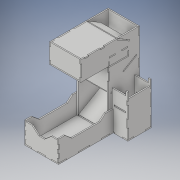
# Autodesk Inventor part: fulltowerv2
Saved by Autodesk Inventor 2017 (Build 210142000, 142)
## iProperties
Created: 2017-03-30
Part Number: fulltowerv2
Material: Generic
Document SubType Name: Modeling
Designer: bearb
Density: 1 g/cm^3
Appearance: Default
Author: bearb
Autodesk Inventor part; units mm, degrees
ref_plane "YZ Plane" through (0, 0, 0) normal (1, 0, 0) x (0, 1, 0)
ref_plane "XZ Plane" through (0, 0, 0) normal (0, 1, 0) x (-1, 0, 0)
ref_plane "XY Plane" through (0, 0, 0) normal (0, 0, 1) x (1, 0, 0)
sketch "Sketch1" plane through (0, 0, 0) normal (1, 0, 0) x (0, 1, 0)
  line L0 (254, 3.81) -> (254, 101.6)
  line L1 (190.5, 101.6) -> (190.5, 34.798)
  line L2 (192.0504, 98.044) -> (212.3704, 98.044) construction
  line L3 (212.3704, 98.044) -> (212.3704, 38.354) construction
  line L4 (212.3704, 38.354) -> (192.0504, 38.354) construction
  line L5 (192.0504, 38.354) -> (192.0504, 98.044) construction
  line L6 (190.5, 101.6) -> (203.2, 101.6)
  line L7 (203.2, 101.6) -> (203.2, 98.044)
  line L8 (203.2, 98.044) -> (190.5, 98.044)
  line L9 (190.5, 98.044) -> (190.5, 101.6)
  line L10 (190.5, 34.798) -> (203.2, 34.798)
  line L11 (203.2, 34.798) -> (203.2, 38.354)
  line L12 (203.2, 38.354) -> (190.5, 38.354)
  line L13 (190.5, 38.354) -> (190.5, 34.798)
  line L14 (190.5, 101.6) -> (186.69, 101.6)
  line L15 (186.69, 101.6) -> (186.69, 34.798)
  line L16 (186.69, 34.798) -> (190.5, 34.798)
  line L17 (212.3704, 38.354) -> (216.1804, 38.354)
  line L18 (216.1804, 38.354) -> (216.1804, 57.404)
  line L19 (216.1804, 57.404) -> (212.3704, 57.404)
  line L20 (212.3704, 57.404) -> (212.3704, 38.354)
  line L21 (212.3704, 98.044) -> (216.1804, 98.044)
  line L22 (216.1804, 98.044) -> (216.1804, 78.994)
  line L23 (216.1804, 78.994) -> (212.3704, 78.994)
  line L24 (212.3704, 78.994) -> (212.3704, 98.044)
  line L25 (231.3686, 31.75) -> (254, 70.9487)
  line L26 (250.9204, 72.7267) -> (228.289, 33.528)
  line L27 (228.289, 33.528) -> (231.3686, 31.75)
  line L28 (254, 70.9487) -> (250.9204, 72.7267)
  line L29 (179.2898, 10.16) -> (153.8898, 54.1541)
  line L30 (153.8898, 54.1541) -> (150.8102, 52.3761)
  line L31 (150.8102, 52.3761) -> (176.2102, 8.382)
  line L32 (176.2102, 8.382) -> (179.2898, 10.16)
  line L33 (114.3, 91.44) -> (85.2445, 41.1145)
  line L34 (85.2445, 41.1145) -> (82.165, 42.8925)
  line L35 (82.165, 42.8925) -> (111.2204, 93.218)
  line L36 (111.2204, 93.218) -> (114.3, 91.44)
  line L37 (9.525, 94.4269) -> (57.15, 11.938)
  line L38 (57.15, 11.938) -> (54.0704, 10.16)
  line L39 (54.0704, 10.16) -> (6.4454, 92.6489)
  line L40 (6.4454, 92.6489) -> (9.525, 94.4269)
  line L41 (254, 177.8) -> (250.19, 177.8)
  line L42 (250.19, 177.8) -> (250.19, 165.1)
  line L43 (250.19, 165.1) -> (254, 165.1)
  line L44 (254, 177.8) -> (254, 190.5)
  line L45 (254, 165.1) -> (254, 127)
  line L46 (254, 127) -> (250.19, 127)
  line L47 (250.19, 127) -> (250.19, 114.3)
  line L48 (250.19, 114.3) -> (254, 114.3)
  line L49 (254, 101.6) -> (254, 114.3)
  line L50 (254, 127) -> (254, 165.1)
  line L51 (228.6, 0) -> (228.6, 3.81)
  line L52 (228.6, 3.81) -> (254, 3.81)
  line L53 (228.6, 0) -> (165.1, 0)
  line L54 (165.1, 0) -> (165.1, 3.81)
  line L55 (165.1, 3.81) -> (139.7, 3.81)
  line L56 (139.7, 3.81) -> (139.7, 0)
  line L57 (139.7, 0) -> (114.3, 0)
  line L58 (114.3, 0) -> (114.3, 3.81)
  line L59 (114.3, 3.81) -> (88.9, 3.81)
  line L60 (88.9, 3.81) -> (88.9, 0)
  line L61 (88.9, 0) -> (50.8, 0)
  line L62 (50.8, 0) -> (50.8, 3.81)
  line L63 (50.8, 3.81) -> (25.4, 3.81)
  line L64 (25.4, 3.81) -> (25.4, 0)
  line L65 (0, 0) -> (25.4, 0)
  line L66 (50.8, 0) -> (88.9, 0)
  line L67 (114.3, 0) -> (139.7, 0)
  line L68 (165.1, 0) -> (228.6, 0)
  line L69 (186.69, 101.6) -> (173.99, 101.6)
  line L70 (173.99, 101.6) -> (173.99, 97.79)
  line L71 (173.99, 97.79) -> (148.59, 97.79)
  line L72 (148.59, 97.79) -> (148.59, 101.6)
  line L73 (190.5, 101.6) -> (173.99, 101.6)
  line L74 (148.59, 101.6) -> (0, 101.6)
  line L75 (0, 101.6) -> (0, 88.9)
  line L76 (0, 0) -> (0, 12.7)
  line L77 (0, 12.7) -> (3.81, 12.7)
  line L78 (0, 88.9) -> (3.81, 88.9)
  line L79 (3.81, 88.9) -> (3.81, 12.7)
  line L80 (0, 101.6) -> (0, 88.9)
  line L81 (0, 12.7) -> (0, 0)
  line L82 (190.5, 190.5) -> (190.5, 177.8)
  line L83 (190.5, 177.8) -> (194.31, 177.8)
  line L84 (194.31, 177.8) -> (194.31, 165.1)
  line L85 (194.31, 165.1) -> (190.5, 165.1)
  line L86 (190.5, 165.1) -> (190.5, 127)
  line L87 (190.5, 127) -> (194.31, 127)
  line L88 (194.31, 127) -> (194.31, 114.3)
  line L89 (194.31, 114.3) -> (190.5, 114.3)
  line L90 (190.5, 101.6) -> (190.5, 114.3)
  line L91 (190.5, 127) -> (190.5, 165.1)
  line L92 (190.5, 177.8) -> (190.5, 190.5)
  line L93 (190.5, 190.5) -> (203.2, 190.5)
  line L94 (203.2, 190.5) -> (203.2, 186.69)
  line L95 (203.2, 186.69) -> (241.3, 186.69)
  line L96 (241.3, 186.69) -> (241.3, 190.5)
  line L97 (190.5, 190.5) -> (203.2, 190.5)
  line L98 (241.3, 190.5) -> (254, 190.5)
  dimension "d0" = 254
  dimension "d2" = 66.802
  dimension "d4" = 20.32
  dimension "d5" = 59.69
  dimension "d6" = 88.9
  dimension "d7" = 12.7
  dimension "d8" = 3.556
  dimension "d9" = 12.7
  dimension "d10" = 3.556
  dimension "d12" = 3.81
  dimension "d13" = 3.81
  dimension "d14" = 19.05
  dimension "d15" = 3.81
  dimension "d16" = 19.05
  dimension "d18" = 3.556
  dimension "d21" = 3.556
  dimension "d22" = 3.556
  dimension "d23" = 3.556
  dimension "d27" = 50.8
  dimension "d30" = 95.25
  dimension "d34" = 3.81
  dimension "d37" = 12.7
  dimension "d38" = 38.1
  dimension "d39" = 3.81
  dimension "d40" = 12.7
  dimension "d43" = 3.81
  dimension "d45" = 3.81
  dimension "d46" = 25.4
  dimension "d47" = 25.4
  dimension "d48" = 25.4
  dimension "d49" = 38.1
  dimension "d50" = 25.4
  dimension "d52" = 12.7
  dimension "d53" = 3.81
  dimension "d54" = 25.4
  dimension "d55" = 12.7
  dimension "d56" = 12.7
  dimension "d57" = 3.81
  dimension "d160" = 12.7
  dimension "d161" = 3.81
  dimension "d162" = 12.7
  dimension "d163" = 38.1
  dimension "d164" = 12.7
  dimension "d165" = 12.7
  dimension "d166" = 3.81
  constraints: 198 end point, 66 perpendicular, 25 parallel, 13 horizontal, 8 point on line, 4 vertical
  measures "d0" distance of L74.end L0.end
  measures "d2" distance of L1.start L1.end
  measures "d4" distance of L3.end L4.end
  measures "d5" distance of L2.end L3.end
  measures "d6" distance of L1.start L82.start
  measures "d7" distance of L7.end L8.end
  measures "d8" distance of L6.end L7.end
  measures "d9" distance of L12.end L11.end
  measures "d10" distance of L11.end L10.end
  measures "d12" distance of L1.start L14.end
  measures "d13" distance of L19.end L18.end
  measures "d14" distance of L18.end L17.end
  measures "d15" distance of L22.end L23.end
  measures "d16" distance of L21.end L22.end
  measures "d18" distance between parallel lines of L26 L25
  measures "d21" distance of L29.end L30.end
  measures "d22" distance of L33.end L34.end
  measures "d23" distance of L37.end L38.end
  measures "d27" distance between parallel lines of L30 L32
  measures "d30" distance between parallel lines of L40 L38
  measures "d34" distance of L43.end L42.end
  measures "d37" distance between parallel lines of L43 L41
  measures "d38" distance of L43.end L45.end
  measures "d39" distance of L45.end L46.end
  measures "d40" distance of L46.end L47.end
  measures "d43" distance of L51.start L51.end
  measures "d45" distance of L53.end L54.end
  measures "d46" distance of L54.end L55.end
  measures "d47" distance of L56.end L57.end
  measures "d48" distance of L58.end L59.end
  measures "d49" distance of L60.end L61.end
  measures "d50" distance of L62.end L63.end
  measures "d52" distance of L14.end L69.end
  measures "d53" distance of L69.end L70.end
  measures "d54" distance of L70.end L71.end
  measures "d55" distance of L74.end L75.end
  measures "d56" distance of L65.start L76.end
  measures "d57" distance of L76.end L77.end
  measures "d160" distance of L82.start L82.end
  measures "d161" distance of L82.end L83.end
  measures "d162" distance of L83.end L84.end
  measures "d163" distance of L85.end L86.end
  measures "d164" distance of L87.end L88.end
  measures "d165" distance of L82.start L93.end
  measures "d166" distance of L93.end L94.end
extrude "Extrusion1" add sketch "Sketch1" along normal blind 3.81 contours L52 L51 L53 L54 L55 L56 L57 L58 L59 L60 L61 L62 L63 L64 L65 L76 L77 L79 L78 L75 L74 L72 L71 L70 L69 L15 L16 L10 L11 L12 L1 L8 L7 L6 L90 L89 L88 L87 L86 L85 L84 L83 L82 L93 L94 L95 L96 L98 L44 L41 L42 L43 L45 L46 L47 L48 L49 L0
sketch "Sketch2" plane through (0, 228.6, 3.81) normal (0, 0, -1) x (-1, 0, 0)
  line L0 (0, 25.4) -> (-3.81, 25.4) projected
  line L1 (0, 25.4) -> (-3.81, 25.4)
  line L2 (0, 0) -> (-3.81, 0) projected
  line L3 (-3.81, 25.4) -> (-3.81, 0)
  line L4 (-3.81, 0) -> (0, 0)
  line L5 (0, 0) -> (0, -63.5)
  line L6 (0, -63.5) -> (-3.81, -63.5) projected
  line L7 (0, -63.5) -> (-3.81, -63.5)
  line L8 (0, -88.9) -> (-3.81, -88.9) projected
  line L9 (-3.81, -63.5) -> (-3.81, -88.9)
  line L10 (-3.81, -88.9) -> (0, -88.9)
  line L11 (0, -88.9) -> (0, -114.3)
  line L12 (0, -114.3) -> (-3.81, -114.3) projected
  line L13 (0, -114.3) -> (-3.81, -114.3)
  line L14 (-3.81, -139.7) -> (-3.81, -114.3) projected
  line L15 (-3.81, -114.3) -> (-3.81, -139.7)
  line L16 (-3.81, -139.7) -> (0, -139.7)
  line L17 (0, -139.7) -> (0, -177.8)
  line L18 (0, -177.8) -> (-3.81, -177.8) projected
  line L19 (0, -177.8) -> (-3.81, -177.8)
  line L20 (-3.81, -177.8) -> (-3.81, -203.2)
  line L21 (0, -203.2) -> (-3.81, -203.2) projected
  line L22 (-3.81, -203.2) -> (0, -203.2)
  line L23 (0, -228.6) -> (-3.81, -228.6) projected
  line L24 (0, -203.2) -> (0, -215.9)
  line L25 (6.35, -228.6) -> (93.98, -228.6)
  line L26 (0, 25.4) -> (-3.81, 25.4) projected
  line L27 (0, 25.4) -> (93.98, 25.4)
  line L28 (93.98, 25.4) -> (97.79, 25.4)
  line L29 (97.79, 25.4) -> (97.79, 0)
  line L30 (97.79, 0) -> (93.98, 0)
  line L31 (93.98, 0) -> (93.98, -63.5)
  line L32 (93.98, -63.5) -> (97.79, -63.5)
  line L33 (97.79, -63.5) -> (97.79, -88.9)
  line L34 (97.79, -88.9) -> (93.98, -88.9)
  line L35 (93.98, -88.9) -> (93.98, -114.3)
  line L36 (93.98, -114.3) -> (97.79, -114.3)
  line L37 (97.79, -114.3) -> (97.79, -139.7)
  line L38 (97.79, -139.7) -> (93.98, -139.7)
  line L39 (93.98, -139.7) -> (93.98, -177.8)
  line L40 (93.98, -177.8) -> (97.79, -177.8)
  line L41 (97.79, -177.8) -> (97.79, -203.2)
  line L42 (97.79, -203.2) -> (93.98, -203.2)
  line L43 (93.98, -203.2) -> (93.98, -228.6)
  line L44 (0, -80.01) -> (0, -228.6) projected
  line L45 (6.35, -228.6) -> (6.35, -215.9)
  line L46 (6.35, -215.9) -> (0, -215.9)
  point P0 (0, -222.25)
  dimension "d62" = 3.81
  dimension "d74" = 93.98
  dimension "d294" = 12.7
  dimension "d295" = 6.35
  constraints: 72 end point, 18 perpendicular, 13 point on line, 6 collinear, 3 horizontal, 1 vertical
  measures "d62" distance of L27.end L28.end
  measures "d74" distance of L0.start L27.end
  measures "d294" distance of L25.start L45.end
  measures "d295" distance of L24.end L45.end
extrude "Extrusion2" add sketch "Sketch2" along normal blind 3.81 separate body contours L27 L28 L29 L30 L31 L32 L33 L34 L35 L36 L37 L38 L39 L40 L41 L42 L43 L25 L45 L46 L24 L44 L17 L11 L8 L9 L6 L5 L2 L3 L0 | L44 L16 L14 L12
ref_plane "Work Plane1" through (-46.99, 0, 0) normal (-1, 0, 0) x (0, 0, 1)
mirror "Mirror1" about plane through (-46.99, 0, 0) normal (-1, 0, 0) bodies 1 separate body
sketch "Sketch5" plane through (-97.79, 54.0704, 10.16) normal (0, 0.8660254, 0.5) x (1, 0, 0)
  line L0 (97.79, 0) -> (101.6, 0) projected
  line L1 (101.6, 0) -> (97.79, 0)
  line L2 (97.79, 0) -> (97.79, 6.35)
  line L3 (97.79, 6.35) -> (3.81, 6.35)
  line L4 (3.81, 6.35) -> (3.81, 0)
  line L5 (3.81, 0) -> (0, 0) projected
  line L6 (3.81, 0) -> (0, 0)
  line L7 (0, 0) -> (0, -95.25)
  line L8 (0, -95.25) -> (3.81, -95.25)
  line L9 (3.81, -95.25) -> (3.81, -101.6)
  line L10 (3.81, -101.6) -> (97.79, -101.6)
  line L11 (97.79, -101.6) -> (97.79, -95.25)
  line L12 (97.79, -95.25) -> (101.6, -95.25) projected
  line L13 (97.79, -95.25) -> (101.6, -95.25)
  line L14 (101.6, 0) -> (101.6, -95.25) projected
  line L15 (101.6, -95.25) -> (101.6, 0)
  dimension "d84" = 6.35
  dimension "d85" = 93.98
  dimension "d86" = 3.81
  dimension "d87" = 6.35
  dimension "d88" = 93.98
  dimension "d89" = 6.35
  dimension "d90" = 3.81
  constraints: 24 end point, 5 perpendicular, 3 point on line, 2 collinear, 1 horizontal
  measures "d84" distance of L0.start L2.end
  measures "d85" distance of L2.end L3.end
  measures "d86" distance of L4.end L5.end
  measures "d87" distance of L8.end L9.end
  measures "d88" distance of L9.end L10.end
  measures "d89" distance of L10.end L11.end
  measures "d90" distance of L11.end L12.end
extrude "Extrusion3" add sketch "Sketch5" along normal blind 3.81 separate body
sketch "Sketch7" plane through (0, 111.2204, 93.218) normal (0, 0.8660254, -0.5) x (1, 0, 0)
  line L0 (3.81, 58.1109) -> (3.81, 0) projected
  line L1 (3.81, 0) -> (3.81, 58.1109)
  line L2 (0, 58.1109) -> (3.81, 58.1109) projected
  line L3 (3.81, 58.1109) -> (0, 58.1109)
  line L4 (0, 0) -> (3.81, 0) projected
  line L5 (3.81, 0) -> (0, 0)
  line L6 (0, 58.1109) -> (0, 64.4609)
  line L7 (0, 64.4609) -> (-93.98, 64.4609)
  line L8 (-97.79, 58.1109) -> (-97.79, 0) projected
  line L9 (-97.79, 58.1109) -> (-97.79, 0)
  line L10 (-97.79, 0) -> (-93.98, 0)
  line L11 (-93.98, 58.1109) -> (-97.79, 58.1109) projected
  line L12 (-97.79, 58.1109) -> (-93.98, 58.1109)
  line L13 (-93.98, 58.1109) -> (-93.98, 64.4609)
  line L14 (0, 0) -> (0, -6.35)
  line L15 (0, -6.35) -> (-93.98, -6.35)
  line L16 (-93.98, -6.35) -> (-93.98, 0)
  point P0 (0, 136.3394)
  dimension "d100" = 3.81
  dimension "d101" = 3.81
  dimension "d102" = 6.35
  dimension "d103" = 93.98
  dimension "d104" = 3.81
  dimension "d105" = 6.35
  dimension "d106" = 93.98
  constraints: 24 end point, 3 collinear, 3 perpendicular, 2 vertical, 1 horizontal
  measures "d100" distance of L0.start L2.start
  measures "d101" distance of L0.end L4.start
  measures "d102" distance of L2.start L6.end
  measures "d103" distance of L6.end L7.end
  measures "d104" distance of L8.end L10.end
  measures "d105" distance of L4.start L14.end
  measures "d106" distance of L14.end L15.end
extrude "Extrusion4" add sketch "Sketch7" along normal blind 3.81 separate body
sketch "Sketch8" plane through (0, 150.8102, 52.3761) normal (0, 0.8660254, 0.5) x (1, 0, 0)
  line L0 (3.81, 50.8) -> (3.81, 0) projected
  line L1 (3.81, 0) -> (3.81, 50.8)
  line L2 (0, 50.8) -> (3.81, 50.8) projected
  line L3 (3.81, 50.8) -> (0, 50.8)
  line L4 (0, 0) -> (3.81, 0) projected
  line L5 (3.81, 0) -> (0, 0)
  line L6 (-97.79, 50.8) -> (-97.79, 0) projected
  line L7 (-97.79, 0) -> (-97.79, 50.8)
  line L8 (-97.79, 50.8) -> (-93.98, 50.8)
  line L9 (-93.98, 0) -> (-97.79, 0) projected
  line L10 (-97.79, 0) -> (-93.98, 0)
  line L11 (0, 50.8) -> (0, 53.34)
  line L12 (0, 53.34) -> (-93.98, 53.34)
  line L13 (-93.98, 53.34) -> (-93.98, 50.8)
  line L14 (0, 0) -> (0, -6.35)
  line L15 (0, -6.35) -> (-93.98, -6.35)
  line L16 (-93.98, -6.35) -> (-93.98, 0)
  point P0 (0, -30.0461)
  dimension "d109" = 3.81
  dimension "d110" = 3.81
  dimension "d111" = 3.81
  dimension "d112" = 3.81
  dimension "d113" = 2.54
  dimension "d114" = 93.98
  dimension "d115" = 6.35
  dimension "d116" = 93.98
  constraints: 24 end point, 3 collinear, 3 perpendicular, 3 vertical, 1 horizontal
  measures "d109" distance of L0.start L2.start
  measures "d110" distance of L0.end L4.start
  measures "d111" distance of L6.start L8.end
  measures "d112" distance of L6.end L9.start
  measures "d113" distance of L2.start L11.end
  measures "d114" distance of L11.end L12.end
  measures "d115" distance of L4.start L14.end
  measures "d116" distance of L14.end L15.end
extrude "Extrusion5" add sketch "Sketch8" along normal blind 3.81 separate body
sketch "Sketch9" plane through (0, 186.69, 101.6) normal (0, 1, 0) x (1, 0, 0)
  line L0 (3.81, 66.802) -> (3.81, 0) projected
  line L1 (0, 66.802) -> (3.81, 66.802) projected
  line L2 (3.81, 0) -> (3.81, 66.802)
  line L3 (3.81, 66.802) -> (-97.79, 66.802)
  line L4 (-93.98, 0) -> (-97.79, 0) projected
  line L5 (-97.79, 66.802) -> (-97.79, 0)
  line L6 (-97.79, 0) -> (3.81, 0)
  point P0 (0, 101.6)
  dimension "d119" = 101.6
  dimension "d120" = 101.6
  constraints: 8 end point, 2 collinear, 1 vertical
  measures "d119" distance of L0.start L3.end
  measures "d120" distance of L4.end L0.end
extrude "Extrusion6" add sketch "Sketch9" along normal blind 3.81 separate body
sketch "Sketch10" plane through (0, 190.5, 98.044) normal (0, 0, 1) x (1, 0, 0)
  line L0 (3.81, 0) -> (3.81, 12.7) projected
  line L1 (3.81, 12.7) -> (3.81, 0)
  line L2 (3.81, 0) -> (-97.79, 0)
  line L3 (0, 0) -> (3.81, 0) projected
  line L4 (-97.79, 0) -> (-97.79, 12.7)
  line L5 (-97.79, 12.7) -> (3.81, 12.7)
  line L6 (-93.98, 12.7) -> (-97.79, 12.7) projected
  point P0 (0, -190.5)
  dimension "d123" = 101.6
  dimension "d124" = 101.6
  constraints: 8 end point, 2 collinear, 1 perpendicular, 1 vertical
  measures "d123" distance of L0.start L2.end
  measures "d124" distance of L4.end L0.end
extrude "Extrusion7" add sketch "Sketch10" along normal blind 3.556 separate body
sketch "Sketch13" plane through (0, 186.69, 34.798) normal (0, 0, 1) x (1, 0, 0)
  line L0 (0, 16.51) -> (3.81, 16.51) projected
  line L1 (3.81, 3.81) -> (-97.79, 3.81) projected
  line L2 (3.81, 3.81) -> (-97.79, 3.81)
  line L3 (-97.79, 3.81) -> (-97.79, 16.51)
  line L4 (-97.79, 16.51) -> (3.81, 16.51)
  line L5 (3.81, 16.51) -> (3.81, 3.81)
  dimension "d136" = 12.7
  dimension "d137" = 101.6
  constraints: 8 end point, 1 collinear, 1 horizontal, 1 perpendicular, 1 point on line, 1 vertical
  measures "d136" distance of L1.end L3.end
  measures "d137" distance of L3.end L0.end
extrude "Extrusion8" add sketch "Sketch13" along normal blind 3.556 separate body
sketch "Sketch14" plane through (0, 212.3704, 57.404) normal (0, 1, 0) x (1, 0, 0)
  line L0 (3.81, 19.05) -> (3.81, 0) projected
  line L1 (3.81, 0) -> (3.81, 19.05)
  line L2 (3.81, 19.05) -> (-97.79, 19.05)
  line L3 (-97.79, 0) -> (-97.79, 19.05) projected
  line L4 (-97.79, 19.05) -> (-97.79, 0)
  line L5 (-97.79, 0) -> (3.81, 0)
  dimension "d140" = 19.05
  dimension "d141" = 101.6
  dimension "d142" = 19.05
  dimension "d143" = 101.6
  constraints: 8 end point, 2 collinear, 2 perpendicular
  measures "d140" distance of L0.end L0.start
  measures "d141" distance of L0.start L2.end
  measures "d142" distance of L2.end L3.start
  measures "d143" distance of L3.start L0.end
extrude "Extrusion9" add sketch "Sketch14" along normal blind 3.81 separate body
sketch "Sketch15" plane through (-97.79, 212.3704, 78.994) normal (0, 1, 0) x (1, 0, 0)
  line L0 (97.79, 0) -> (101.6, 0)
  line L1 (3.81, -19.05) -> (0, -19.05)
  line L2 (101.6, 0) -> (101.6, -19.05)
  line L3 (101.6, 0) -> (101.6, -19.05)
  line L4 (101.6, -19.05) -> (0, -19.05)
  line L5 (0, 0) -> (101.6, 0)
  line L6 (3.81, 0) -> (0, 0)
  line L7 (0, 0) -> (0, -19.05)
  line L8 (0, 0) -> (0, -19.05)
  dimension "d146" = 19.05
  dimension "d147" = 101.6
  dimension "d148" = 19.05
  dimension "d150" = 101.6
  dimension "d151" = 101.6
  constraints: 18 end point
  measures "d146" distance of L2.end L0.end
  measures "d147" distance of L0.end L5.start
  measures "d148" distance of L5.start L1.end
  measures "d150" distance of L2.end L1.end
  measures "d151" distance of L5.start L0.end
extrude "Extrusion10" add sketch "Sketch15" along normal blind 3.81 separate body
sketch "Sketch16" plane through (-97.79, 228.289, 33.528) normal (0, 0.8660254, -0.5) x (1, 0, 0)
  line L0 (0, 0) -> (0, -45.2627) projected
  line L1 (0, 0) -> (0, -45.2627)
  line L2 (0, -45.2627) -> (101.6, -45.2627)
  line L3 (101.6, -45.2627) -> (101.6, 0)
  line L4 (97.79, 0) -> (101.6, 0) projected
  line L5 (101.6, 0) -> (97.79, 0)
  line L6 (97.79, 0) -> (97.79, 2.54)
  line L7 (97.79, 2.54) -> (0, 2.54)
  line L8 (3.81, 2.54) -> (3.81, 0)
  line L9 (3.81, 0) -> (0, 0) projected
  line L10 (3.81, 0) -> (0, 0)
  dimension "d154" = 101.6
  dimension "d155" = 3.81
  dimension "d156" = 2.54
  dimension "d157" = 97.79
  constraints: 16 end point, 3 perpendicular, 2 collinear, 1 horizontal, 1 point on line, 1 vertical
  measures "d154" distance of L0.end L2.end
  measures "d155" distance of L3.end L4.start
  measures "d156" distance of L4.start L6.end
  measures "d157" distance of L6.end L7.end
extrude "Extrusion11" add sketch "Sketch16" along normal blind 3.81 separate body
sketch "Sketch17" plane through (0, 194.31, 165.1) normal (0, -1, 0) x (1, 0, 0)
  line L0 (3.81, 0) -> (3.81, 12.7) projected
  line L1 (3.81, 12.7) -> (3.81, 0)
  line L2 (0, 0) -> (3.81, 0) projected
  line L3 (3.81, 0) -> (0, 0)
  line L4 (0, 0) -> (0, -38.1)
  line L5 (0, -38.1) -> (3.81, -38.1) projected
  line L6 (0, -38.1) -> (3.81, -38.1)
  line L7 (3.81, -38.1) -> (3.81, -50.8)
  line L8 (0, -50.8) -> (3.81, -50.8) projected
  line L9 (3.81, -50.8) -> (0, -50.8)
  line L10 (-93.98, -63.5) -> (-93.98, -50.8)
  line L11 (-93.98, -50.8) -> (-97.79, -50.8)
  line L12 (-97.79, -38.1) -> (-97.79, -50.8) projected
  line L13 (-97.79, -50.8) -> (-97.79, -38.1)
  line L14 (-97.79, -38.1) -> (-93.98, -38.1)
  line L15 (-93.98, -38.1) -> (-93.98, 0)
  line L16 (-93.98, 0) -> (-97.79, 0)
  line L17 (-97.79, 0) -> (-97.79, 12.7)
  line L18 (-93.98, 12.7) -> (-97.79, 12.7) projected
  line L19 (-97.79, 12.7) -> (-93.98, 12.7)
  line L20 (-93.98, 12.7) -> (-93.98, 25.4)
  line L21 (-93.98, 25.4) -> (0, 25.4)
  line L22 (0, 12.7) -> (3.81, 12.7) projected
  line L23 (3.81, 12.7) -> (0, 12.7)
  line L24 (0, 12.7) -> (0, 25.4)
  line L25 (0, -50.8) -> (0, -63.5)
  line L26 (0, -63.5) -> (-93.98, -63.5)
  line L27 (-53.34, 22.86) -> (-40.64, 22.86)
  line L28 (-40.64, 22.86) -> (-40.64, 5.08)
  line L29 (-40.64, 5.08) -> (-53.34, 5.08)
  line L30 (-53.34, 5.08) -> (-53.34, 22.86)
  dimension "d168" = 93.98
  dimension "d169" = 3.81
  dimension "d170" = 12.7
  dimension "d171" = 93.98
  dimension "d172" = 68.58
  dimension "d173" = 17.78
  dimension "d174" = 12.7
  dimension "d175" = 40.64
  constraints: 48 end point, 10 perpendicular, 6 equal length, 6 point on line, 1 horizontal, 1 vertical
  measures "d168" distance of L25.end L10.start
  measures "d169" distance of L10.end L11.end
  measures "d170" distance of L11.end L12.start
  measures "d171" distance of L20.end L21.end
  measures "d172" distance between parallel lines of L26 L29
  measures "d173" distance between parallel lines of L27 L29
  measures "d174" distance between parallel lines of L28 L30
  measures "d175" distance from line of L21.end L28
extrude "Extrusion12" add sketch "Sketch17" along normal blind 3.81 bodies 1
sketch "Sketch18" plane through (-93.98, 203.2, 186.69) normal (0, 0, 1) x (1, 0, 0)
  line L0 (-3.81, 38.1) -> (-3.81, 0) projected
  line L1 (-3.81, 0) -> (-3.81, 38.1)
  line L2 (-3.81, 38.1) -> (0, 38.1)
  line L3 (0, 38.1) -> (0, 50.8)
  line L4 (0, 50.8) -> (93.98, 50.8)
  line L5 (93.98, 50.8) -> (93.98, 38.1)
  line L6 (93.98, 38.1) -> (97.79, 38.1) projected
  line L7 (93.98, 38.1) -> (97.79, 38.1)
  line L8 (97.79, 38.1) -> (97.79, 0) projected
  line L9 (97.79, 38.1) -> (97.79, 0)
  line L10 (97.79, 0) -> (93.98, 0)
  line L11 (93.98, 0) -> (93.98, -8.89)
  line L12 (93.98, -8.89) -> (0, -8.89)
  line L13 (0, -8.89) -> (0, 0)
  line L14 (0, 0) -> (-3.81, 0) projected
  line L15 (0, 0) -> (-3.81, 0)
  dimension "d178" = 38.1
  dimension "d179" = 3.81
  dimension "d180" = 12.7
  dimension "d181" = 93.98
  dimension "d182" = 38.1
  dimension "d184" = 8.89
  dimension "d185" = 93.98
  constraints: 24 end point, 5 perpendicular, 2 collinear, 2 vertical, 1 horizontal
  measures "d178" distance of L0.end L0.start
  measures "d179" distance of L0.start L2.end
  measures "d180" distance of L2.end L3.end
  measures "d181" distance of L3.end L4.end
  measures "d182" distance of L6.end L8.end
  measures "d184" distance of L10.end L11.end
  measures "d185" distance of L11.end L12.end
extrude "Extrusion13" add sketch "Sketch18" along normal blind 3.81 separate body
sketch "Sketch19" plane through (-93.98, 250.19, 127) normal (0, 1, 0) x (1, 0, 0)
  line L0 (97.79, 12.7) -> (93.98, 12.7)
  line L1 (93.98, 12.7) -> (93.98, 53.848)
  line L2 (93.98, 53.848) -> (0, 53.848)
  line L3 (0, 53.848) -> (0, 12.7)
  line L4 (0, 12.7) -> (-3.81, 12.7)
  line L5 (-3.81, 12.7) -> (-3.81, 0)
  line L6 (-3.81, 0) -> (0, 0)
  line L7 (0, 0) -> (0, -38.1)
  line L8 (0, -38.1) -> (-3.81, -38.1)
  line L9 (-3.81, -38.1) -> (-3.81, -50.8)
  line L10 (0, -50.8) -> (-3.81, -50.8)
  line L11 (-3.81, -50.8) -> (0, -50.8)
  line L12 (0, -50.8) -> (0, -59.69)
  line L13 (0, -59.69) -> (93.98, -59.69)
  line L14 (93.98, -59.69) -> (93.98, -50.8)
  line L15 (93.98, -50.8) -> (97.79, -50.8)
  line L16 (97.79, -50.8) -> (97.79, -38.1)
  line L17 (97.79, -38.1) -> (93.98, -38.1)
  line L18 (93.98, -38.1) -> (93.98, 0)
  line L19 (93.98, 0) -> (97.79, 0)
  line L20 (97.79, 12.7) -> (97.79, 0)
  line L21 (97.79, 0) -> (97.79, 12.7)
  line L22 (93.98, 12.7) -> (97.79, 12.7)
  line L23 (97.79, 12.7) -> (93.98, 12.7)
  dimension "d188" = 41.148
  dimension "d189" = 93.98
  dimension "d190" = 38.1
  dimension "d191" = 8.89
  dimension "d192" = 93.98
  constraints: 48 end point, 1 point on line
  measures "d188" distance of L0.end L1.end
  measures "d189" distance of L1.end L2.end
  measures "d190" distance of L6.end L7.end
  measures "d191" distance of L10.start L12.end
  measures "d192" distance of L12.end L13.end
extrude "Extrusion14" add sketch "Sketch19" along normal blind 3.81 separate body
sketch "Sketch20" plane through (0, 148.59, 97.79) normal (0, 0, 1) x (1, 0, 0)
  line L0 (3.81, 25.4) -> (3.81, 0) projected
  line L1 (3.81, 0) -> (3.81, 25.4)
  line L2 (3.81, 25.4) -> (0, 25.4)
  line L3 (0, 25.4) -> (0, 41.91)
  line L4 (0, 41.91) -> (-93.98, 41.91)
  line L5 (-93.98, 25.4) -> (-97.79, 25.4) projected
  line L6 (-93.98, 41.91) -> (-93.98, 25.4)
  line L7 (-93.98, 25.4) -> (-97.79, 25.4)
  line L8 (-97.79, 25.4) -> (-97.79, 0)
  line L9 (-93.98, 0) -> (-97.79, 0) projected
  line L10 (-97.79, 0) -> (-93.98, 0)
  line L11 (-93.98, 0) -> (-93.98, -29.21)
  line L12 (-93.98, -29.21) -> (0, -29.21)
  line L13 (0, -29.21) -> (0, 0)
  line L14 (0, 0) -> (3.81, 0)
  dimension "d195" = 3.81
  dimension "d196" = 16.51
  dimension "d197" = 93.98
  dimension "d198" = 29.21
  dimension "d199" = 93.98
  constraints: 24 end point, 5 perpendicular, 3 collinear, 1 vertical
  measures "d195" distance of L0.start L2.end
  measures "d196" distance of L2.end L3.end
  measures "d197" distance of L3.end L4.end
  measures "d198" distance of L9.start L11.end
  measures "d199" distance of L11.end L12.end
extrude "Extrusion15" add sketch "Sketch20" along normal blind 3.81 separate body
sketch "Sketch21" plane through (0, 3.81, 12.7) normal (0, -1, 0) x (1, 0, 0)
  line L0 (0, 0) -> (3.81, 0) projected
  line L1 (0, 76.2) -> (3.81, 76.2) projected
  line L2 (3.81, 76.2) -> (0, 76.2)
  line L3 (0, 88.9) -> (0, 76.2) projected
  line L4 (0, 76.2) -> (0, 88.9)
  line L5 (0, 88.9) -> (-93.98, 88.9)
  line L6 (-93.98, 87.3532) -> (0, 87.3532) projected
  line L7 (-93.98, 88.9) -> (-93.98, 76.2) projected
  line L8 (-93.98, 88.9) -> (-93.98, 76.2)
  line L9 (-93.98, 76.2) -> (-97.79, 76.2) projected
  line L10 (-93.98, 76.2) -> (-97.79, 76.2)
  line L11 (-97.79, 76.2) -> (-97.79, 0)
  line L12 (-93.98, 0) -> (-97.79, 0) projected
  line L13 (-97.79, 0) -> (-93.98, 0)
  line L14 (3.81, 0) -> (0, 0)
  line L15 (0, 0) -> (0, -8.89)
  line L16 (0, -8.89) -> (-93.98, -8.89)
  line L17 (-93.98, 0) -> (-93.98, -8.89)
  line L18 (0, 76.2) -> (12.7, 76.2)
  line L19 (12.7, 76.2) -> (12.7, 72.39)
  line L20 (12.7, 72.39) -> (38.1, 72.39)
  line L21 (38.1, 72.39) -> (38.1, 76.2)
  line L22 (0, 0) -> (12.7, 0)
  line L23 (12.7, 0) -> (12.7, 3.81)
  line L24 (12.7, 3.81) -> (38.1, 3.81)
  line L25 (38.1, 3.81) -> (38.1, 0)
  line L26 (0, 0) -> (12.7, 0)
  line L27 (38.1, 0) -> (54.61, 0)
  line L28 (54.61, 76.2) -> (38.1, 76.2)
  line L29 (12.7, 76.2) -> (0, 76.2)
  line L30 (54.61, 76.2) -> (54.61, 57.15)
  line L31 (54.61, 57.15) -> (50.8, 57.15)
  line L32 (54.61, 0) -> (54.61, 19.05)
  line L33 (54.61, 19.05) -> (50.8, 19.05)
  line L34 (50.8, 19.05) -> (50.8, 57.15)
  line L35 (54.61, 0) -> (54.61, 19.05)
  line L36 (54.61, 57.15) -> (54.61, 76.2)
  dimension "d204" = 8.89
  dimension "d205" = 93.98
  dimension "d206" = 54.61
  dimension "d207" = 76.2
  dimension "d208" = 12.7
  dimension "d209" = 3.81
  dimension "d210" = 25.4
  dimension "d211" = 12.7
  dimension "d212" = 3.81
  dimension "d213" = 25.4
  dimension "d214" = 19.05
  dimension "d215" = 3.81
  dimension "d216" = 19.05
  dimension "d217" = 3.81
  constraints: 60 end point, 14 perpendicular, 4 collinear, 3 parallel, 2 horizontal, 2 vertical
  measures "d204" distance of L0.start L15.end
  measures "d205" distance of L15.end L16.end
  measures "d206" distance of L0.start L27.end
  measures "d207" distance of L27.end L28.start
  measures "d208" distance of L1.start L18.end
  measures "d209" distance of L18.end L19.end
  measures "d210" distance of L19.end L20.end
  measures "d211" distance of L0.start L22.end
  measures "d212" distance of L22.end L23.end
  measures "d213" distance of L23.end L24.end
  measures "d214" distance of L28.start L30.end
  measures "d215" distance of L30.end L31.end
  measures "d216" distance of L27.end L32.end
  measures "d217" distance of L32.end L33.end
extrude "Extrusion16" add sketch "Sketch21" along normal blind 3.81 separate body
sketch "Sketch22" plane through (12.7, 3.81, 85.09) normal (0, 0, 1) x (1, 0, 0)
  line L0 (0, 0) -> (-8.89, 0)
  line L1 (-12.7, 0) -> (0, 0) projected
  line L2 (0, 0) -> (0, -3.81)
  line L3 (0, -3.81) -> (25.4, -3.81) projected
  line L4 (0, -3.81) -> (25.4, -3.81)
  line L5 (25.4, 0) -> (25.4, -3.81) projected
  line L6 (25.4, -3.81) -> (25.4, 0)
  line L7 (41.91, 0) -> (38.1, 0) projected
  line L8 (25.4, 0) -> (41.91, 0)
  line L9 (41.91, 133.35) -> (35.56, 133.35)
  line L10 (35.56, 133.35) -> (35.56, 120.65)
  line L11 (35.56, 120.65) -> (-8.89, 120.65)
  line L12 (-8.89, 110.49) -> (-8.89, 135.89) projected
  line L13 (-8.89, 120.65) -> (-8.89, 0)
  line L14 (-2.54, 76.5265) -> (35.56, 76.5265)
  line L15 (35.56, 76.5265) -> (35.56, 72.7165)
  line L16 (35.56, 72.7165) -> (-2.54, 72.7165)
  line L17 (-2.54, 72.7165) -> (-2.54, 76.5265)
  line L18 (41.91, 133.35) -> (41.91, 107.95)
  line L19 (41.91, 107.95) -> (38.1, 107.95)
  line L20 (38.1, 107.95) -> (38.1, 95.25)
  line L21 (38.1, 95.25) -> (41.91, 95.25)
  line L22 (41.91, 95.25) -> (41.91, 57.15)
  line L23 (41.91, 57.15) -> (38.1, 57.15)
  line L24 (38.1, 57.15) -> (38.1, 31.75)
  line L25 (38.1, 31.75) -> (41.91, 31.75)
  line L26 (41.91, 0) -> (41.91, 31.75)
  line L27 (41.91, 57.15) -> (41.91, 95.25)
  line L28 (41.91, 107.95) -> (41.91, 133.35)
  dimension "d220" = 8.89
  dimension "d221" = 133.35
  dimension "d222" = 6.35
  dimension "d223" = 12.7
  dimension "d224" = 38.1
  dimension "d225" = 3.81
  dimension "d227" = 25.4
  dimension "d228" = 3.81
  dimension "d229" = 12.7
  dimension "d230" = 38.1
  dimension "d231" = 3.81
  dimension "d232" = 25.4
  constraints: 48 end point, 16 perpendicular, 4 point on line, 3 collinear, 2 horizontal, 2 parallel, 1 vertical
  measures "d220" distance of L0.start L0.end
  measures "d221" distance of L7.start L9.start
  measures "d222" distance of L9.start L9.end
  measures "d223" distance of L9.end L10.end
  measures "d224" distance of L15.end L16.end
  measures "d225" distance of L14.end L15.end
  measures "d227" distance of L9.start L18.end
  measures "d228" distance of L18.end L19.end
  measures "d229" distance of L19.end L20.end
  measures "d230" distance of L21.end L22.end
  measures "d231" distance of L22.end L23.end
  measures "d232" distance of L23.end L24.end
extrude "Extrusion17" add sketch "Sketch22" along normal blind 3.81 separate body
ref_plane "Work Plane2" through (12.7, 3.81, 50.8) normal (0, 0, -1) x (-1, 0, 0)
mirror "Mirror2" about plane through (12.7, 3.81, 50.8) normal (0, 0, -1) bodies 17
sketch "Sketch23" plane through (50.8, 99.06, 85.09) normal (1, 0, 0) x (0, 0, -1)
  line L0 (-3.81, 0) -> (-3.81, 12.7)
  line L1 (-3.81, 0) -> (-3.81, 12.7)
  line L2 (-3.81, 12.7) -> (0, 12.7)
  line L3 (0, 12.7) -> (0, 19.05)
  line L4 (0, 19.05) -> (68.58, 19.05)
  line L5 (68.58, 19.05) -> (68.58, 12.7)
  line L6 (68.58, 12.7) -> (72.39, 12.7)
  line L7 (68.58, 12.7) -> (72.39, 12.7)
  line L8 (72.39, 12.7) -> (72.39, 0)
  line L9 (68.58, 0) -> (72.39, 0)
  line L10 (72.39, 0) -> (68.58, 0)
  line L11 (68.58, 0) -> (68.58, -38.1)
  line L12 (68.58, -38.1) -> (72.39, -38.1)
  line L13 (68.58, -38.1) -> (72.39, -38.1)
  line L14 (72.39, -63.5) -> (72.39, -38.1)
  line L15 (72.39, -38.1) -> (72.39, -63.5)
  line L16 (72.39, -63.5) -> (68.58, -63.5)
  line L17 (68.58, -63.5) -> (68.58, -95.25)
  line L18 (68.58, -95.25) -> (53.34, -95.25)
  line L19 (53.34, -95.25) -> (53.34, -99.06)
  line L20 (53.34, -99.06) -> (15.24, -99.06)
  line L21 (53.34, -99.06) -> (15.24, -99.06)
  line L22 (15.24, -99.06) -> (15.24, -95.25)
  line L23 (15.24, -95.25) -> (0, -95.25)
  line L24 (0, -95.25) -> (0, -63.5)
  line L25 (0, -63.5) -> (-3.81, -63.5)
  line L26 (0, -63.5) -> (-3.81, -63.5)
  line L27 (-3.81, -63.5) -> (-3.81, -38.1)
  line L28 (0, -38.1) -> (0, 0)
  line L29 (-3.81, -38.1) -> (0, -38.1)
  line L30 (0, -38.1) -> (0, 0)
  line L31 (0, 0) -> (-3.81, 0) projected
  line L32 (0, 0) -> (-3.81, 0)
  line L33 (-3.81, 0) -> (0, 0)
  dimension "d238" = 12.7
  dimension "d239" = 3.81
  dimension "d240" = 6.35
  dimension "d241" = 68.58
  dimension "d242" = 3.81
  dimension "d243" = 3.81
  dimension "d244" = 31.75
  dimension "d245" = 3.81
  dimension "d246" = 38.1
  dimension "d247" = 25.4
  constraints: 66 end point, 2 point on line, 1 collinear, 1 horizontal
  measures "d238" distance of L0.start L0.end
  measures "d239" distance of L0.end L2.end
  measures "d240" distance of L2.end L3.end
  measures "d241" distance of L3.end L4.end
  measures "d242" distance of L5.end L6.end
  measures "d243" distance of L11.end L12.end
  measures "d244" distance of L16.end L17.end
  measures "d245" distance of L18.end L19.end
  measures "d246" distance of L19.end L20.end
  measures "d247" distance of L25.end L27.end
extrude "Extrusion18" add sketch "Sketch23" along normal blind 3.81 separate body
sketch "Sketch24" plane through (-97.79, 0, 101.6) normal (-1, 0, 0) x (0, 0, 1)
  line L0 (-12.7, 3.81) -> (-12.7, 0)
  line L1 (-12.7, 67.31) -> (-12.7, 3.81)
  line L2 (0, 3.81) -> (25.4, 3.81)
  line L3 (25.4, 3.81) -> (25.4, 0)
  line L4 (25.4, 0) -> (63.5, 0)
  line L5 (63.5, 0) -> (63.5, 3.81)
  line L6 (63.5, 3.81) -> (101.6, 3.81)
  line L7 (101.6, 3.81) -> (101.6, 0)
  line L8 (101.6, 0) -> (139.7, 0)
  line L9 (139.7, 0) -> (139.7, 3.81)
  line L10 (165.1, 3.81) -> (139.7, 3.81)
  line L11 (25.4, 0) -> (63.5, 0)
  line L12 (101.6, 0) -> (139.7, 0)
  line L13 (101.6, 3.81) -> (63.5, 3.81)
  line L14 (25.4, 3.81) -> (0, 3.81)
  line L15 (-12.7, 67.31) -> (12.7, 67.31)
  line L16 (12.7, 67.31) -> (30.7715, 52.1462)
  line L17 (30.7715, 52.1462) -> (121.6285, 52.1462)
  line L18 (121.6285, 52.1462) -> (144.3314, 71.1962)
  line L19 (165.1, 71.1962) -> (144.3314, 71.1962)
  line L20 (12.7, 67.31) -> (-12.7, 67.31)
  line L21 (-12.7, 0) -> (0, 0)
  line L22 (0, 0) -> (0, 3.81)
  line L23 (165.1, 3.81) -> (165.1, 16.51)
  line L24 (165.1, 16.51) -> (161.296, 16.51)
  line L25 (161.296, 16.51) -> (161.296, 29.21)
  line L26 (161.296, 29.21) -> (165.1, 29.21)
  line L27 (165.1, 29.21) -> (165.1, 41.91)
  line L28 (165.1, 41.91) -> (161.296, 41.91)
  line L29 (161.296, 41.91) -> (161.296, 54.61)
  line L30 (161.296, 54.61) -> (165.1, 54.61)
  line L31 (165.1, 54.61) -> (165.1, 71.1962)
  line L32 (165.1, 3.81) -> (165.1, 16.51)
  line L33 (165.1, 29.21) -> (165.1, 41.91)
  dimension "d256" = 38.1
  dimension "d257" = 38.1
  dimension "d258" = 38.1
  dimension "d263" = 12.7
  dimension "d264" = 12.7
  dimension "d265" = 12.7
  dimension "d266" = 12.7
  dimension "d276" = 19.05
  constraints: 68 end point, 10 perpendicular, 2 point on line, 1 horizontal
  measures "d256" distance of L3.end L4.end
  measures "d257" distance of L5.end L6.end
  measures "d258" distance of L8.end L7.end
  measures "d263" distance of L10.start L23.end
  measures "d264" distance of L24.end L25.end
  measures "d265" distance of L26.end L27.end
  measures "d266" distance of L28.end L29.end
  measures "d276" distance between parallel lines of L19 L17
extrude "Extrusion19" add sketch "Sketch24" along normal blind 3.81 separate body
ref_plane "Work Plane3" through (-46.99, 0, 101.6) normal (1, 0, 0) x (0, 0, -1)
mirror "Mirror3" about plane through (-46.99, 0, 101.6) normal (1, 0, 0) bodies 19
sketch "Sketch25" plane through (-97.79, 41.91, 262.896) normal (0, 0, 1) x (1, 0, 0)
  line L0 (-3.81, 0) -> (-3.81, 12.7)
  line L1 (-3.81, 12.7) -> (0, 12.7)
  line L2 (0, 12.7) -> (0, 25.4)
  line L3 (101.6, 25.4) -> (101.6, 12.7)
  line L4 (101.6, 12.7) -> (105.41, 12.7)
  line L5 (105.41, 12.7) -> (105.41, 0)
  line L6 (101.6, 0) -> (105.41, 0)
  line L7 (101.6, 0) -> (101.6, -12.7)
  line L8 (101.6, -12.7) -> (105.41, -12.7)
  line L9 (105.41, -12.7) -> (105.41, -25.4)
  line L10 (105.41, -25.4) -> (101.6, -25.4)
  line L11 (0, -38.1) -> (0, -25.4)
  line L12 (0, -25.4) -> (-3.81, -25.4)
  line L13 (-3.81, -25.4) -> (-3.81, -12.7)
  line L14 (-3.81, -12.7) -> (0, -12.7)
  line L15 (0, 0) -> (-3.81, 0)
  line L16 (0, 25.4) -> (19.05, 25.4)
  line L17 (19.05, 25.4) -> (41.7529, 6.35)
  line L18 (41.7529, 6.35) -> (59.8471, 6.35)
  line L19 (59.8471, 6.35) -> (82.55, 25.4)
  line L20 (0, 25.4) -> (19.05, 25.4)
  line L21 (82.55, 25.4) -> (101.6, 25.4)
  line L22 (19.05, -38.1) -> (19.05, -41.91)
  line L23 (38.1, -41.91) -> (38.1, -38.1)
  line L24 (82.55, -41.91) -> (82.55, -38.1)
  line L25 (63.5, -38.1) -> (63.5, -41.91)
  line L26 (101.6, -25.4) -> (101.6, -38.1)
  line L27 (82.55, -41.91) -> (63.5, -41.91)
  line L28 (38.1, -41.91) -> (19.05, -41.91)
  line L29 (19.05, -38.1) -> (0, -38.1)
  line L30 (82.55, -38.1) -> (101.6, -38.1)
  line L31 (38.1, -38.1) -> (63.5, -38.1)
  line L32 (0, -12.7) -> (0, 0)
  dimension "d270" = 3.81
  dimension "d271" = 12.7
  dimension "d272" = 12.7
  dimension "d274" = 19.05
  dimension "d275" = 19.05
  dimension "d282" = 19.05
  constraints: 66 end point, 3 point on line, 1 horizontal, 1 vertical
  measures "d270" distance of L0.end L1.end
  measures "d271" distance of L6.start L7.end
  measures "d272" distance of L8.end L9.end
  measures "d274" distance of L2.end L16.end
  measures "d275" distance of L3.start L19.end
  measures "d282" distance from line of L2.end L18
extrude "Extrusion20" add sketch "Sketch25" along normal blind 3.81 separate body
sketch "Sketch26" plane through (3.81, 3.81, 165.1) normal (0, -1, 0) x (1, 0, 0)
  line L0 (3.81, 0) -> (3.81, 38.1) projected
  line L1 (3.81, -0.0008) -> (3.81, 38.1)
  line L2 (3.81, 38.1) -> (0, 38.1)
  line L3 (0, 38.1) -> (0, 76.2)
  line L4 (0, 76.2) -> (3.81, 76.2)
  line L5 (3.81, 76.2) -> (3.81, 101.6) projected
  line L6 (3.81, 76.2) -> (3.81, 101.6)
  line L7 (3.81, 101.6) -> (-19.05, 101.606)
  line L8 (-19.05, 101.606) -> (-19.051, 97.791)
  line L9 (-19.051, 97.791) -> (-38.1, 97.796)
  line L10 (-38.1, 97.796) -> (-38.099, 101.6111)
  line L11 (-63.5, 101.606) -> (-38.1, 101.606) projected
  line L12 (-38.099, 101.6111) -> (-63.5, 101.606)
  line L13 (-63.5, 97.796) -> (-63.5, 101.606) projected
  line L14 (-63.5, 101.606) -> (-63.5, 97.796)
  line L15 (-82.55, 97.796) -> (-82.55, 101.606) projected
  line L16 (-63.5, 97.796) -> (-82.55, 97.796)
  line L17 (-82.55, 97.796) -> (-82.55, 101.606)
  line L18 (-82.55, 101.606) -> (-105.41, 101.6)
  line L19 (-105.41, 76.2) -> (-105.41, 101.6) projected
  line L20 (-105.41, 101.6) -> (-105.41, 76.2)
  line L21 (-101.6, 76.2) -> (-105.41, 76.2) projected
  line L22 (-105.41, 76.2) -> (-101.6, 76.2)
  line L23 (-101.6, 38.1) -> (-105.41, 38.1) projected
  line L24 (-101.6, 76.2) -> (-101.6, 38.1)
  line L25 (-101.6, 38.1) -> (-105.41, 38.1)
  line L26 (-105.41, 0) -> (-105.41, 38.1) projected
  line L27 (-105.41, 38.1) -> (-105.41, 0)
  line L28 (-105.41, 0) -> (-101.6, 0)
  line L29 (-101.6, 0) -> (-101.6, -38.1)
  line L30 (-105.41, -63.5) -> (-105.41, -38.1) projected
  line L31 (-101.6, -38.1) -> (-105.41, -38.1)
  line L32 (-105.41, -38.1) -> (-105.41, -63.5)
  line L33 (-105.41, -63.5) -> (-101.6, -63.5)
  line L34 (3.81, -63.5) -> (3.81, -38.1) projected
  line L35 (-101.6, -63.5) -> (3.81, -63.5)
  line L36 (3.81, -63.5) -> (3.81, -38.1)
  line L37 (3.81, -38.1) -> (0, -38.1)
  line L38 (0, -38.1) -> (0, 0)
  line L39 (0, 0) -> (3.81, 0) projected
  line L40 (3.81, 0) -> (0, 0)
  dimension "d289" = 3.81
  constraints: 58 end point, 19 perpendicular, 5 collinear, 3 point on line
  measures "d289" distance of L0.end L2.end
extrude "Extrusion21" add sketch "Sketch26" along normal blind 3.81 separate body
body "Solid1"
body "Solid2"
body "Solid3"
body "Solid4"
body "Solid5"
body "Solid6"
body "Solid7"
body "Solid8"
body "Solid9"
body "Solid10"
body "Solid11"
body "Solid12"
body "Solid13"
body "Solid14"
body "Solid15"
body "Solid16"
body "Solid17"
body "Solid18"
body "Solid19"
body "Solid20"
body "Solid21"
